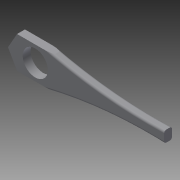
# Autodesk Inventor part: Leg
Saved by Autodesk Inventor 2015 (Build 190159000, 159)
## iProperties
Created: 2016-04-24
Part Number: Leg
Material: Generic
Document SubType Name: Modeling
Designer: Hatch
Density: 1 g/cm^3
Appearance: Default
Author: Hatch
Autodesk Inventor part; units mm, degrees
ref_plane "YZ Plane" through (0, 0, 0) normal (1, 0, 0) x (0, 1, 0)
ref_plane "XZ Plane" through (0, 0, 0) normal (0, 1, 0) x (-1, 0, 0)
ref_plane "XY Plane" through (0, 0, 0) normal (0, 0, 1) x (1, 0, 0)
sketch "Sketch1" plane through (0, 0, 0) normal (0, 1, 0) x (-1, 0, 0)
  circle A0 centre (0, 0) radius 11.125
  line L0 (0, -11.125) -> (0, -14.125)
  line L1 (0, 11.125) -> (0, 14.125)
  line L2 (11.125, 0) -> (16.125, 0)
  line L3 (16.125, 14.125) -> (-113.875, 14.125)
  line L4 (-113.875, 14.125) -> (-113.875, -14.125)
  line L5 (-113.875, -14.125) -> (16.125, -14.125)
  line L6 (16.125, -14.125) -> (16.125, 14.125)
  dimension "d0" = 22.25
  dimension "d1" = 3
  dimension "d2" = 3
  dimension "d3" = 5
  dimension "d6" = 130
  constraints: 14 end point, 3 point on circle, 2 horizontal, 2 parallel, 2 vertical, 1 centre point, 1 coincident, 1 midpoint, 1 perpendicular
  measures "d0" diameter of A0
  measures "d1" distance of L0.start L0.end
  measures "d2" distance of L1.start L1.end
  measures "d3" distance of L2.end L2.start
  measures "d6" distance of L5.end L4.end
extrude "Extrusion1" add sketch "Sketch1" along normal blind 7 contours L2 L6 L5 L0 A0 | A0 L1 L3 L6 L2 | A0 L0 L5 L4 L3 L1
sketch "Sketch2" plane through (0, 0, 0) normal (0, -1, 0) x (1, 0, 0)
  line L0 (113.875, 14.125) -> (113.875, -14.125) projected
  line L1 (113.875, 0) -> (113.875, 5)
  line L2 (113.875, 5) -> (113.875, -5)
  circle A0 centre (0, 0) radius 11.125 projected
  line L3 (11.125, 0) -> (16.125, 0)
  line L4 (-16.125, 14.125) -> (113.875, 14.125) projected
  line L5 (16.125, 14.125) -> (16.125, -14.125)
  line L6 (113.875, -14.125) -> (-16.125, -14.125) projected
  arc A1 (16.125, 14.125) -> (113.875, 5) centre (100.0237, 384.7475) ccw
  arc A2 (113.875, -5) -> (16.125, -14.125) centre (100.0237, -384.7475) ccw
  line L7 (16.125, 14.125) -> (113.875, 14.125)
  line L8 (113.875, 14.125) -> (113.875, 5)
  line L9 (16.125, -14.125) -> (113.875, -14.125)
  line L10 (113.875, -14.125) -> (113.875, -5)
  dimension "d9" = 5
  dimension "d10" = 10
  dimension "d11" = 5
  dimension "d12" = 380
  dimension "d13" = 380
  constraints: 16 end point, 4 collinear, 4 point on circle, 4 point on line, 2 centre point, 1 horizontal, 1 horizontal alignment, 1 midpoint, 1 vertical, 1 other
  measures "d9" distance of L1.start L1.end
  measures "d10" distance of L1.end L2.end
  measures "d11" distance of L3.start L3.end
  measures "d12" radius of A1
  measures "d13" radius of A2
extrude "Extrusion2" cut sketch "Sketch2" against normal through all contours L0 A1 L4 | L0 L6 A2
fillet "Fillet1" radius 2 1 edges at (64.7041, 0, 6.3924)
fillet "Fillet2" radius 2 1 edges at (64.7041, 7, 6.3924)
fillet "Fillet3" radius 2 1 edges at (64.7041, 0, -6.3924)
fillet "Fillet4" radius 2 1 edges at (64.7041, 7, -6.3924)
sketch "Sketch3" plane through (0, 0, 0) normal (0, -1, 0) x (1, 0, 0)
  line L0 (-16.125, -14.125) -> (-16.125, 14.125) projected
  line L1 (-16.125, 0) -> (-24.125, 0)
  line L2 (-24.125, 0) -> (-16.125, 14.125)
  line L3 (-16.125, 14.125) -> (-16.125, -14.125)
  line L4 (-16.125, -14.125) -> (-24.125, 0)
  point P0 (0, 0)
  dimension "d20" = 8
  constraints: 8 end point, 1 collinear, 1 horizontal, 1 midpoint
  measures "d20" distance of L1.start L1.end
extrude "Extrusion3" add sketch "Sketch3" against normal blind 7
body "Solid1"
